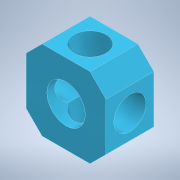
# Autodesk Inventor part: nut
Saved by Autodesk Inventor 2022 (Build 260153000, 153)
## iProperties
Created: 2023-03-07
Part Number: nut
Material: Generic
Document SubType Name: Modeling
Designer: karee
Density: 1 g/cm^3
Appearance: Turquoise
Author: karee
Autodesk Inventor part; units mm, degrees
ref_plane "YZ Plane" through (0, 0, 0) normal (1, 0, 0) x (0, 1, 0)
ref_plane "XZ Plane" through (0, 0, 0) normal (0, 1, 0) x (-1, 0, 0)
ref_plane "XY Plane" through (0, 0, 0) normal (0, 0, 1) x (1, 0, 0)
sketch "Sketch1" plane through (0, 0, 0) normal (0, 0, 1) x (1, 0, 0)
  point P0 (0, 0)
sketch "Sketch2" plane through (0, 0, 0) normal (0, 0, 1) x (1, 0, 0)
  line L0 (0, 0) -> (25, 0)
  line L1 (25, 0) -> (25, 25)
  line L2 (25, 25) -> (0, 25)
  line L3 (0, 25) -> (0, 0)
  dimension "d0" = 25
  dimension "d1" = 25
  constraints: 8 end point, 2 parallel, 1 horizontal, 1 perpendicular
  measures "d0" distance of L2.end L1.end
  measures "d1" distance of L1.end L0.end
extrude "Extrusion1" add sketch "Sketch2" along normal blind 15
chamfer "Chamfer1" distance 5 angle 45 4 edges at (25, 25, 7.5) (25, 0, 7.5) (0, 25, 7.5) (0, 0, 7.5)
sketch "Sketch3" plane through (0, 0, 15) normal (0, 0, 1) x (1, 0, 0)
  line L0 (20, 25) -> (5, 25) projected
  circle A0 centre (12.5, 12.5) radius 6
  line L1 (25, 5) -> (25, 20) projected
  point P0 (0, 0)
  dimension "d7" = 12
  dimension "d8" = 12.5
  dimension "d9" = 12.5
  constraints: 1 centre point
  measures "d7" diameter of A0
  measures "d8" distance from line of A0.centre L0
  measures "d9" distance from line of A0.centre L1
extrude "Extrusion2" cut sketch "Sketch3" against normal blind 15
sketch "Sketch4" plane through (0, 5, 0) normal (-1, 0, 0) x (0, 0, 1)
  circle A0 centre (7.5, 7.5) radius 5.05
  line L0 (15, 20) -> (0, 20) projected
  line L1 (15, 15) -> (15, 0) projected
  point P0 (0, -5)
  dimension "d12" = 10.1
  dimension "d13" = 12.5
  dimension "d14" = 7.5
  constraints: 1 centre point
  measures "d12" diameter of A0
  measures "d13" distance from line of A0.centre L0
  measures "d14" distance from line of A0.centre L1
extrude "Extrusion3" cut sketch "Sketch4" against normal through all
sketch "Sketch5" plane through (5, 25, 0) normal (0, 1, 0) x (1, 0, 0)
  circle A0 centre (7.5, -7.5) radius 5.05
  line L0 (15, 0) -> (0, 0) projected
  line L1 (-5, 0) -> (-5, -15) projected
  dimension "d17" = 10.1
  dimension "d18" = 7.5
  dimension "d19" = 12.5
  constraints: 1 centre point
  measures "d17" diameter of A0
  measures "d18" distance from line of A0.centre L0
  measures "d19" distance from line of A0.centre L1
extrude "Extrusion4" cut sketch "Sketch5" against normal through all
body "Solid1"
